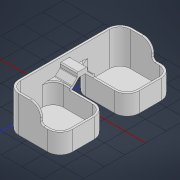
# Autodesk Inventor part: Purge_Bucket
Saved by Autodesk Inventor 2022 (Build 260153000, 153)
## iProperties
Created: 2022-03-02
Part Number: Purge_Bucket
Material: Generisch
Document SubType Name: Modeling
Designer: sleib
Density: 1 g/cm^3
Appearance: Vorgabe
Author: sleib
Autodesk Inventor part; units mm, degrees
ref_plane "YZ Plane" through (0, 0, 0) normal (1, 0, 0) x (0, 1, 0)
ref_plane "XZ Plane" through (0, 0, 0) normal (0, 1, 0) x (-1, 0, 0)
ref_plane "XY Plane" through (0, 0, 0) normal (0, 0, 1) x (1, 0, 0)
sketch "Skizze1" plane through (0, 0, 0) normal (0, 1, 0) x (-1, 0, 0)
  line L0 (-12, 55) -> (-40, 55)
  line L1 (-52, 43) -> (-52, 22)
  line L2 (-40, 10) -> (-12, 10)
  line L3 (0, 22) -> (0, 43)
  line L4 (13.8794, 0) -> (-65.8794, 0) construction
  line L5 (0, -80.4794) -> (0, 80.4794) construction
  arc A0 (0, 43) -> (-12, 55) centre (-12, 43) ccw
  arc A1 (-12, 10) -> (0, 22) centre (-12, 22) ccw
  arc A2 (-52, 22) -> (-40, 10) centre (-40, 22) ccw
  arc A3 (-40, 55) -> (-52, 43) centre (-40, 43) ccw
  line L6 (-40, 53) -> (-12, 53)
  arc A4 (-2, 43) -> (-12, 53) centre (-12, 43) ccw
  line L7 (-2, 43) -> (-2, 22)
  arc A5 (-12, 12) -> (-2, 22) centre (-12, 22) ccw
  line L8 (-12, 12) -> (-40, 12)
  arc A6 (-50, 22) -> (-40, 12) centre (-40, 22) ccw
  line L9 (-50, 22) -> (-50, 43)
  arc A7 (-40, 53) -> (-50, 43) centre (-40, 43) ccw
  line L10 (0, 22) -> (0, 0)
  line L11 (0, 22) -> (-2, 22)
  line L12 (-2, 22) -> (-2, 0)
  line L13 (-40, 53) -> (-40, 55)
  line L14 (-12, -55) -> (-40, -55)
  line L15 (-52, -43) -> (-52, -22)
  line L16 (-40, -10) -> (-12, -10)
  line L17 (0, -22) -> (0, -43)
  arc A8 (-12, -55) -> (0, -43) centre (-12, -43) ccw
  arc A9 (0, -22) -> (-12, -10) centre (-12, -22) ccw
  arc A10 (-40, -10) -> (-52, -22) centre (-40, -22) ccw
  arc A11 (-52, -43) -> (-40, -55) centre (-40, -43) ccw
  line L18 (-40, -53) -> (-12, -53)
  arc A12 (-12, -53) -> (-2, -43) centre (-12, -43) ccw
  line L19 (-2, -43) -> (-2, -22)
  arc A13 (-2, -22) -> (-12, -12) centre (-12, -22) ccw
  line L20 (-12, -12) -> (-40, -12)
  arc A14 (-40, -12) -> (-50, -22) centre (-40, -22) ccw
  line L21 (-50, -22) -> (-50, -43)
  arc A15 (-50, -43) -> (-40, -53) centre (-40, -43) ccw
  line L22 (0, -22) -> (0, 0)
  line L23 (0, -22) -> (-2, -22)
  line L24 (-2, -22) -> (-2, 0)
  line L25 (-40, -53) -> (-40, -55)
  point P0 (0, 55)
  point P1 (-52, 10)
  point P2 (-52, 55)
  point P3 (-2.4, 14.8)
  point P4 (0, -55)
  point P5 (-52, -10)
  point P6 (-52, -55)
  point P7 (-2.4, -14.8)
  dimension "d0" = 45
  dimension "d2" = 10
  dimension "d3" = 52
  dimension "d4" = 12
  dimension "d5" = 2
  constraints: 48 end point, 34 point on circle, 24 symmetric about line, 16 centre point, 13 point on line, 10 tangent, 4 parallel, 3 equal radius, 3 perpendicular, 2 collinear, 2 vertical, 1 horizontal, 15 other
  measures "d0" distance of point (-52, 55) point (-52, 10)
  measures "d2" distance between parallel lines of L2 L4
  measures "d3" distance of point (0, 55) point (-52, 55)
  measures "d4" radius of A0
  measures "d5" distance between parallel lines of L0 L6
extrude "Extrusion1" add sketch "Skizze1" against normal blind 19 contours A0 L3 L11 L7 A4 L6 L13 L0 | L13 A7 L9 A6 L8 A5 L12 A1 L2 A2 L1 A3 | L6 A4 L7 A5 L8 A6 L9 A7 | A1 L12 L11 | L23 L24 A9 | L17 A8 L14 L25 L18 A12 L19 L23 | L24 A13 L20 A14 L21 A15 L25 A11 L15 A10 L16 A9 | L19 A12 L18 A15 L21 A14 L20 A13
extrude "Extrusion8" cut sketch "Skizze1" against normal blind 17 contours L6 A4 L7 A5 L8 A6 L9 A7 | L19 A12 L18 A15 L21 A14 L20 A13
extrude "Extrusion2" add sketch "Skizze1" along normal blind 16 contours A0 L3 L11 L7 A4 L6 L13 L0 | L10 L22 A9 L24 L12 A1 | A1 L12 L11 | L23 L24 A9 | L17 A8 L14 L25 L18 A12 L19 L23
sketch "Skizze3" plane through (0, -19, 22) normal (-1, 0, 0) x (0, 0, 1)
  line L0 (-22, 19) -> (-22, 35) construction
  line L1 (21, 35) -> (-65, 35) projected
  line L2 (-25, 26) -> (-19, 26)
  line L3 (-44, 19) -> (0, 19) projected
  line L4 (-44, 19) -> (-37.3668, 19) projected
  line L5 (-44, 19) -> (-44, 0) projected
  line L6 (-32, 0) -> (-44, 0) projected
  line L7 (-32, 19) -> (-32, 0) projected
  line L8 (-37.3668, 19) -> (-32, 19) projected
  line L9 (-12, 19) -> (-6.6332, 19) projected
  line L10 (-12, 19) -> (-12, 0) projected
  line L11 (0, 0) -> (-12, 0) projected
  line L12 (0, 19) -> (0, 0) projected
  line L13 (-6.6332, 19) -> (0, 19) projected
  line L14 (-25, 26) -> (-44, 7)
  line L15 (-19, 26) -> (0, 7)
  line L16 (-44, 19) -> (-44, 0) projected
  line L17 (-44, 7) -> (-44, 19)
  line L18 (-44, 19) -> (-32, 19)
  line L19 (0, 19) -> (-12, 19) projected
  line L20 (-12, 19) -> (0, 19)
  line L21 (0, 19) -> (0, 7)
  line L22 (-27, 31) -> (-17, 31)
  line L23 (-27, 31) -> (-27, 26.8284)
  line L24 (-27, 26.8284) -> (-32, 21.8284)
  line L25 (-17, 31) -> (-17, 26.8284)
  line L26 (-17, 26.8284) -> (-12, 21.8284)
  line L27 (-32, 21.8284) -> (-34, 21.8284)
  line L28 (-34, 21.8284) -> (-34, 19)
  line L29 (-6.6332, 19) -> (-37.3668, 19) projected
  line L30 (-32, 19) -> (-34, 19)
  line L31 (-12, 21.8284) -> (-10, 21.8284)
  line L32 (-10, 21.8284) -> (-10, 19)
  line L33 (-12, 19) -> (-10, 19)
  line L34 (-34, 19) -> (-34, 2) projected
  line L35 (-34, 19) -> (-34, 2) projected
  line L36 (-10, 19) -> (-10, 2) projected
  line L37 (-10, 19) -> (-10, 2) projected
  point P0 (-22, 26)
  point P1 (-22, 31)
  point P2 (-12, 19)
  dimension "d19" = 6
  dimension "d21" = 135
  dimension "d22" = 5
  dimension "d23" = 2
  dimension "d24" = 2
  dimension "d27" = 10
  dimension "d48" = 7
  constraints: 38 end point, 7 point on line, 6 perpendicular, 4 collinear, 4 horizontal, 3 midpoint, 3 vertical, 2 parallel, 2 vertical alignment
  measures "d19" distance of L2.start L2.end
  measures "d21" angle of L2 L14
  measures "d22" distance between parallel lines of L2 L22
  measures "d23" distance between parallel lines of L14 L24
  measures "d24" distance between parallel lines of L15 L26
  measures "d27" distance between parallel lines of L25 L23
  measures "d48" distance between parallel lines of L3 L2
extrude "Extrusion5" add sketch "Skizze3" against normal blind 18.5 contours L14 L3 L28 L27 L24 L23 L22 L25 L26 L31 L32 L15 L2
extrude "Extrusion6" add sketch "Skizze3" against normal up to next contours L14 L34 L3 | L3 L36 L15 | L34 L14 L5 L3 | L3 L12 L15 L36
extrude "Extrusion7" cut sketch "Skizze3" against normal through all contours L2 L15 L3 L14
sketch "Skizze4" plane through (0, 0, 0) normal (0, 1, 0) x (1, 0, 0)
  arc A0 (12, -12) -> (2, -22) centre (12, -22) ccw projected
  line L0 (2, -12) -> (12, -12) projected
  line L1 (2, -12) -> (2, -22) projected
  arc A1 (2, 22) -> (12, 12) centre (12, 22) ccw projected
  line L2 (2, 12) -> (2, 22) projected
  line L3 (2, 12) -> (12, 12) projected
  point P0 (0, 0)
extrude "Extrusion9" add sketch "Skizze4" along normal up to surface (2.8284 mm away)
sketch "Skizze5" plane through (12, -19, 55) normal (0, 0, 1) x (1, 0, 0)
  line L0 (-12, 0) -> (-12, 35) projected
  line L1 (0, 35) -> (-12, 35) projected
  line L2 (0, 35) -> (28, 35) projected
  line L3 (28, 19) -> (28, 35) projected
  line L4 (28, 19) -> (28, 0) projected
  line L5 (28, 0) -> (0, 0) projected
  line L6 (-12, 0) -> (0, 0) projected
  arc A0 (21, 25) -> (11, 35) centre (11, 25) ccw
  arc A1 (21, 22) -> (24, 19) centre (24, 22) ccw
  line L7 (21, 25) -> (21, 22)
  line L8 (28, 19) -> (28, 2) projected
  line L9 (28, 19) -> (24, 19)
  line L10 (11, 35) -> (28, 35)
  line L11 (28, 19) -> (28, 35) projected
  line L12 (28, 19) -> (28, 35)
  point P0 (-12, 19)
  dimension "d38" = 33
  dimension "d39" = 10
  dimension "d40" = 3
  constraints: 8 end point, 5 tangent, 4 point on circle, 2 centre point, 2 collinear, 1 horizontal, 1 point on line, 1 vertical
  measures "d38" distance between parallel lines of L7 L0
  measures "d39" radius of A0
  measures "d40" radius of A1
extrude "Extrusion10" cut sketch "Skizze5" against normal through all contours L2 L3 L9 A1 L7 A0
fillet "Rundung1" radius 1 10 edges at (10.25, 12, 5) (10.25, 12, -5) (10.25, 2.8284, -10) (10.25, 2.8284, 10) (15.25, 2.8284, 12) (4.9289, 2.8284, 14.9289) (15.25, 2.8284, -12) (4.9289, 2.8284, -14.9289) (10.25, 7.8284, -5) (10.25, 7.8284, 5)
sketch "Skizze6" plane through (0, 7, -3) normal (0, -1, 0) x (1, 0, 0)
  line L0 (18.5, 6) -> (18.5, 0) projected
  line L1 (18.5, 3) -> (0, 3) construction
  circle A0 centre (13.25, 3) radius 3
  circle A1 centre (5.25, 3) radius 3
  line L2 (0, 6) -> (18.5, 6) projected
  line L3 (9.25, 6) -> (9.25, 0) construction
  line L4 (0, 0) -> (18.5, 0) projected
  dimension "d45" = 8
  constraints: 4 end point, 3 midpoint, 2 centre point, 2 point on line, 2 tangent, 1 horizontal, 1 symmetric about line
  measures "d45" distance of A1.centre A0.centre
extrude "Extrusion11" cut sketch "Skizze6" against normal blind 3 contours A0 | A1
